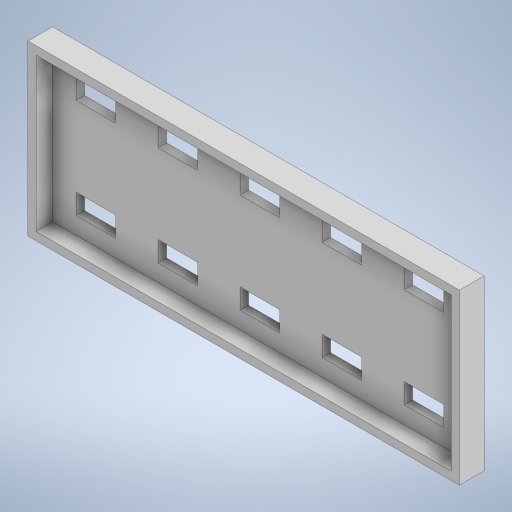
# Autodesk Inventor part: RelayCaseTop
Saved by Autodesk Inventor 2024 (Build 280153000, 153)
## iProperties
Created: 2023-08-11
Part Number: RelayCaseTop
Material: Generic
Document SubType Name: Modeling
Designer: 18179
Density: 1 g/cm^3
Appearance: Default
Autodesk Inventor part; units mm, degrees
ref_plane "YZ Plane" through (0, 0, 0) normal (1, 0, 0) x (0, 1, 0)
ref_plane "XZ Plane" through (0, 0, 0) normal (0, 1, 0) x (-1, 0, 0)
ref_plane "XY Plane" through (0, 0, 0) normal (0, 0, 1) x (1, 0, 0)
sketch "0" plane through (0, 0, 0) normal (0, 0, 1) x (1, 0, 0)
  line L0 (-191.1389, 47.736) -> (-191.1389, -4.588)
  line L1 (-191.1389, -4.588) -> (-185.2969, -4.588)
  line L2 (-185.2969, -4.588) -> (-170.0569, -4.588)
  line L3 (-170.0569, -4.588) -> (-153.5469, -4.588)
  line L4 (-153.5469, -4.588) -> (-138.3069, -4.588)
  line L5 (-138.3069, -4.588) -> (-121.7969, -4.588)
  line L6 (-121.7969, -4.588) -> (-106.5569, -4.588)
  line L7 (-106.5569, -4.588) -> (-90.0469, -4.588)
  line L8 (-90.0469, -4.588) -> (-74.8069, -4.588)
  line L9 (-74.8069, -4.588) -> (-58.2969, -4.588)
  line L10 (-58.2969, -4.588) -> (-43.0569, -4.588)
  line L11 (-43.0569, -4.588) -> (-37.2149, -4.588)
  line L12 (-37.2149, -4.588) -> (-37.2149, 47.736)
  line L13 (-37.2149, 47.736) -> (-43.0569, 47.736)
  line L14 (-43.0569, 47.736) -> (-58.2969, 47.736)
  line L15 (-58.2969, 47.736) -> (-74.8069, 47.736)
  line L16 (-74.8069, 47.736) -> (-90.0469, 47.736)
  line L17 (-90.0469, 47.736) -> (-106.5569, 47.736)
  line L18 (-106.5569, 47.736) -> (-121.7969, 47.736)
  line L19 (-121.7969, 47.736) -> (-138.3069, 47.736)
  line L20 (-138.3069, 47.736) -> (-153.5469, 47.736)
  line L21 (-153.5469, 47.736) -> (-170.0569, 47.736)
  line L22 (-170.0569, 47.736) -> (-185.2969, 47.736)
  line L23 (-185.2969, 47.736) -> (-191.1389, 47.736)
  line L24 (-90.0469, -1.159) -> (-90.0469, 6.588)
  line L25 (-90.0469, 6.588) -> (-90.0215, 6.588)
  line L26 (-90.0215, 6.588) -> (-90.0215, 24.368)
  line L27 (-90.0215, 24.368) -> (-74.8323, 24.368)
  line L28 (-74.8323, 24.368) -> (-74.8323, 6.588)
  line L29 (-74.8323, 6.588) -> (-74.8069, 6.588)
  line L30 (-74.8069, 6.588) -> (-74.8069, -1.159)
  line L31 (-74.8069, -1.159) -> (-90.0469, -1.159)
  line L32 (-74.8069, 37.449) -> (-90.0469, 37.449)
  line L33 (-90.0469, 37.449) -> (-90.0469, 45.196)
  line L34 (-90.0469, 45.196) -> (-74.8069, 45.196)
  line L35 (-74.8069, 45.196) -> (-74.8069, 37.449)
  line L36 (-153.5469, -1.159) -> (-153.5469, 6.588)
  line L37 (-153.5469, 6.588) -> (-153.5215, 6.588)
  line L38 (-153.5215, 6.588) -> (-153.5215, 24.368)
  line L39 (-153.5215, 24.368) -> (-138.3323, 24.368)
  line L40 (-138.3323, 24.368) -> (-138.3323, 6.588)
  line L41 (-138.3323, 6.588) -> (-138.3069, 6.588)
  line L42 (-138.3069, 6.588) -> (-138.3069, -1.159)
  line L43 (-138.3069, -1.159) -> (-153.5469, -1.159)
  line L44 (-138.3069, 37.449) -> (-153.5469, 37.449)
  line L45 (-153.5469, 37.449) -> (-153.5469, 45.196)
  line L46 (-153.5469, 45.196) -> (-138.3069, 45.196)
  line L47 (-138.3069, 45.196) -> (-138.3069, 37.449)
  line L48 (-185.2969, -1.159) -> (-185.2969, 6.588)
  line L49 (-185.2969, 6.588) -> (-185.2715, 6.588)
  line L50 (-185.2715, 6.588) -> (-185.2715, 24.368)
  line L51 (-185.2715, 24.368) -> (-170.0823, 24.368)
  line L52 (-170.0823, 24.368) -> (-170.0823, 6.588)
  line L53 (-170.0823, 6.588) -> (-170.0569, 6.588)
  line L54 (-170.0569, 6.588) -> (-170.0569, -1.159)
  line L55 (-170.0569, -1.159) -> (-185.2969, -1.159)
  line L56 (-170.0569, 37.449) -> (-185.2969, 37.449)
  line L57 (-185.2969, 37.449) -> (-185.2969, 45.196)
  line L58 (-185.2969, 45.196) -> (-170.0569, 45.196)
  line L59 (-170.0569, 45.196) -> (-170.0569, 37.449)
  line L60 (-106.5569, 37.449) -> (-121.7969, 37.449)
  line L61 (-121.7969, 37.449) -> (-121.7969, 45.196)
  line L62 (-121.7969, 45.196) -> (-106.5569, 45.196)
  line L63 (-106.5569, 45.196) -> (-106.5569, 37.449)
  line L64 (-121.7969, -1.159) -> (-121.7969, 6.588)
  line L65 (-121.7969, 6.588) -> (-121.7715, 6.588)
  line L66 (-121.7715, 6.588) -> (-121.7715, 24.368)
  line L67 (-121.7715, 24.368) -> (-106.5823, 24.368)
  line L68 (-106.5823, 24.368) -> (-106.5823, 6.588)
  line L69 (-106.5823, 6.588) -> (-106.5569, 6.588)
  line L70 (-106.5569, 6.588) -> (-106.5569, -1.159)
  line L71 (-106.5569, -1.159) -> (-121.7969, -1.159)
  line L72 (-58.2715, 6.588) -> (-58.2715, 24.368)
  line L73 (-58.2715, 24.368) -> (-43.0823, 24.368)
  line L74 (-43.0823, 24.368) -> (-43.0823, 6.588)
  line L75 (-43.0823, 6.588) -> (-43.0569, 6.588)
  line L76 (-43.0569, 6.588) -> (-43.0569, -1.159)
  line L77 (-43.0569, -1.159) -> (-58.2969, -1.159)
  line L78 (-58.2969, -1.159) -> (-58.2969, 6.588)
  line L79 (-58.2969, 6.588) -> (-58.2715, 6.588)
  line L80 (-58.2969, 37.449) -> (-58.2969, 45.196)
  line L81 (-58.2969, 45.196) -> (-43.0569, 45.196)
  line L82 (-43.0569, 45.196) -> (-43.0569, 37.449)
  line L83 (-43.0569, 37.449) -> (-58.2969, 37.449)
  line L84 (-34.0399, 50.911) -> (-194.3139, 50.911)
  line L85 (-194.3139, -7.763) -> (-34.0399, -7.763)
  line L86 (-34.0399, -7.763) -> (-34.0399, 50.911)
  line L87 (-191.1389, 47.736) -> (-37.2149, 47.736)
  line L88 (-37.2149, 47.736) -> (-37.2149, -4.588)
  line L89 (-37.2149, -4.588) -> (-191.1389, -4.588)
  line L90 (-191.1389, -4.588) -> (-191.1389, 47.736)
  circle A0 centre (-92.4599, 44.3888) radius 1.524
  circle A1 centre (-72.3939, 44.3888) radius 1.524
  circle A2 centre (-92.4599, -1.2407) radius 1.524
  circle A3 centre (-72.3939, -1.2407) radius 1.524
  circle A4 centre (-155.9599, 44.3888) radius 1.524
  circle A5 centre (-135.8939, 44.3888) radius 1.524
  circle A6 centre (-155.9599, -1.2407) radius 1.524
  circle A7 centre (-135.8939, -1.2407) radius 1.524
  circle A8 centre (-187.7099, 44.3888) radius 1.524
  circle A9 centre (-167.6439, 44.3888) radius 1.524
  circle A10 centre (-187.7099, -1.2407) radius 1.524
  circle A11 centre (-167.6439, -1.2407) radius 1.524
  circle A12 centre (-104.1439, -1.2407) radius 1.524
  circle A13 centre (-124.2099, -1.2407) radius 1.524
  circle A14 centre (-104.1439, 44.3888) radius 1.524
  circle A15 centre (-124.2099, 44.3888) radius 1.524
  circle A16 centre (-40.6439, 44.3888) radius 1.524
  circle A17 centre (-60.7099, 44.3888) radius 1.524
  circle A18 centre (-40.6439, -1.2407) radius 1.524
  circle A19 centre (-60.7099, -1.2407) radius 1.524
  line L91 (-194.3139, 50.911) -> (-34.0399, 50.911)
  line L92 (-34.0399, 50.911) -> (-34.0399, -7.763)
  line L93 (-34.0399, -7.763) -> (-194.3139, -7.763)
  line L94 (-194.3139, -7.763) -> (-194.3139, 50.911)
  line L95 (-194.5189, 51.1161) -> (-33.8348, 51.1161)
  line L96 (-33.8348, 51.1161) -> (-33.8348, -7.968)
  line L97 (-33.8348, -7.968) -> (-194.5189, -7.968)
  line L98 (-194.5189, -7.968) -> (-194.5189, 51.1161)
  line L99 (-197.6939, 54.2911) -> (-30.6598, 54.2911)
  line L100 (-30.6598, 54.2911) -> (-30.6598, -11.143)
  line L101 (-30.6598, -11.143) -> (-197.6939, -11.143)
  line L102 (-197.6939, -11.143) -> (-197.6939, 54.2911)
  point P0 (-43.0569, -1.159)
  point P1 (-106.5823, 6.588)
  point P2 (-106.5569, -1.159)
  point P3 (-170.0823, 6.588)
  point P4 (-170.0569, -1.159)
  point P5 (-138.3323, 6.588)
  point P6 (-138.3069, -1.159)
  point P7 (-74.8323, 6.588)
  point P8 (-74.8069, -1.159)
  dimension "d0" = 3.175
  constraints: 206 end point, 20 centre point, 6 parallel, 3 perpendicular, 1 horizontal, 6 other
  measures "d0" distance between parallel lines of L98 L102
extrude "Extrusion1" add sketch "0" along normal blind 6.35 contours L99 L100 L101 L102
extrude "Extrusion2" add sketch "0" against normal blind 3.175 contours L23 L22 L21 L20 L19 L18 L17 L16 L15 L14 L13 L12 L11 L10 L9 L8 L7 L6 L5 L4 L3 L2 L1 L0 | L86 L85 L94 L84 | A0 | A1 | A2 | A3 | A4 | A5 | A6 | A7 | A8 | A9 | A10 | A11 | A12 | A13 | A14 | A15 | A16 | A17 | A18 | A19 | L95 L96 L97 L98 | L99 L100 L101 L102
sketch "Sketch3" plane through (0, 0, 0) normal (0, 0, 1) x (1, 0, 0)
  line L0 (-43.0569, -1.159) -> (-43.0569, 6.588) projected
  line L1 (-185.2969, 6.588) -> (-185.2969, -1.159) projected
  line L2 (-43.0569, 6.588) -> (-185.2969, 6.588)
  line L3 (-90.0469, -1.159) -> (-90.0469, 6.588) projected
  line L4 (-90.0469, 6.588) -> (-90.0215, 6.588) projected
  line L5 (-90.0215, 6.588) -> (-90.0215, 24.368) projected
  line L6 (-90.0215, 24.368) -> (-74.8323, 24.368) projected
  line L7 (-74.8323, 24.368) -> (-74.8323, 6.588) projected
  line L8 (-74.8323, 6.588) -> (-74.8069, 6.588) projected
  line L9 (-74.8069, 6.588) -> (-74.8069, -1.159) projected
  line L10 (-74.8069, -1.159) -> (-90.0469, -1.159) projected
  line L11 (-74.8069, 37.449) -> (-90.0469, 37.449) projected
  line L12 (-90.0469, 37.449) -> (-90.0469, 45.196) projected
  line L13 (-90.0469, 45.196) -> (-74.8069, 45.196) projected
  line L14 (-74.8069, 45.196) -> (-74.8069, 37.449) projected
  line L15 (-153.5469, -1.159) -> (-153.5469, 6.588) projected
  line L16 (-153.5469, 6.588) -> (-153.5215, 6.588) projected
  line L17 (-153.5215, 6.588) -> (-153.5215, 24.368) projected
  line L18 (-153.5215, 24.368) -> (-138.3323, 24.368) projected
  line L19 (-138.3323, 24.368) -> (-138.3323, 6.588) projected
  line L20 (-138.3323, 6.588) -> (-138.3069, 6.588) projected
  line L21 (-138.3069, 6.588) -> (-138.3069, -1.159) projected
  line L22 (-138.3069, -1.159) -> (-153.5469, -1.159) projected
  line L23 (-138.3069, 37.449) -> (-153.5469, 37.449) projected
  line L24 (-153.5469, 37.449) -> (-153.5469, 45.196) projected
  line L25 (-153.5469, 45.196) -> (-138.3069, 45.196) projected
  line L26 (-138.3069, 45.196) -> (-138.3069, 37.449) projected
  line L27 (-185.2969, -1.159) -> (-185.2969, 6.588) projected
  line L28 (-185.2969, 6.588) -> (-185.2715, 6.588) projected
  line L29 (-185.2715, 6.588) -> (-185.2715, 24.368) projected
  line L30 (-185.2715, 24.368) -> (-170.0823, 24.368) projected
  line L31 (-170.0823, 24.368) -> (-170.0823, 6.588) projected
  line L32 (-170.0823, 6.588) -> (-170.0569, 6.588) projected
  line L33 (-170.0569, 6.588) -> (-170.0569, -1.159) projected
  line L34 (-170.0569, -1.159) -> (-185.2969, -1.159) projected
  line L35 (-170.0569, 37.449) -> (-185.2969, 37.449) projected
  line L36 (-185.2969, 37.449) -> (-185.2969, 45.196) projected
  line L37 (-185.2969, 45.196) -> (-170.0569, 45.196) projected
  line L38 (-170.0569, 45.196) -> (-170.0569, 37.449) projected
  line L39 (-106.5569, 37.449) -> (-121.7969, 37.449) projected
  line L40 (-121.7969, 37.449) -> (-121.7969, 45.196) projected
  line L41 (-121.7969, 45.196) -> (-106.5569, 45.196) projected
  line L42 (-106.5569, 45.196) -> (-106.5569, 37.449) projected
  line L43 (-121.7969, -1.159) -> (-121.7969, 6.588) projected
  line L44 (-121.7969, 6.588) -> (-121.7715, 6.588) projected
  line L45 (-121.7715, 6.588) -> (-121.7715, 24.368) projected
  line L46 (-121.7715, 24.368) -> (-106.5823, 24.368) projected
  line L47 (-106.5823, 24.368) -> (-106.5823, 6.588) projected
  line L48 (-106.5823, 6.588) -> (-106.5569, 6.588) projected
  line L49 (-106.5569, 6.588) -> (-106.5569, -1.159) projected
  line L50 (-106.5569, -1.159) -> (-121.7969, -1.159) projected
  line L51 (-58.2715, 6.588) -> (-58.2715, 24.368) projected
  line L52 (-58.2715, 24.368) -> (-43.0823, 24.368) projected
  line L53 (-43.0823, 24.368) -> (-43.0823, 6.588) projected
  line L54 (-43.0823, 6.588) -> (-43.0569, 6.588) projected
  line L55 (-43.0569, 6.588) -> (-43.0569, -1.159) projected
  line L56 (-43.0569, -1.159) -> (-58.2969, -1.159) projected
  line L57 (-58.2969, -1.159) -> (-58.2969, 6.588) projected
  line L58 (-58.2969, 6.588) -> (-58.2715, 6.588) projected
  line L59 (-58.2969, 37.449) -> (-58.2969, 45.196) projected
  line L60 (-58.2969, 45.196) -> (-43.0569, 45.196) projected
  line L61 (-43.0569, 45.196) -> (-43.0569, 37.449) projected
  line L62 (-43.0569, 37.449) -> (-58.2969, 37.449) projected
  line L63 (-194.5189, -7.968) -> (-194.5189, 51.1161) projected
  line L64 (-33.8348, -7.968) -> (-194.5189, -7.968) projected
  line L65 (-33.8348, 51.1161) -> (-33.8348, -7.968) projected
  line L66 (-194.5189, 51.1161) -> (-33.8348, 51.1161) projected
  point P0 (0, 0)
  constraints: 2 end point, 1 horizontal
extrude "Extrusion3" add sketch "Sketch3" against normal blind 3.175 contours L2 L51 L52 L53 | L29 L30 L31 L2 | L2 L5 L6 L7 | L2 L45 L46 L47 | L2 L17 L18 L19
body "Solid1"
